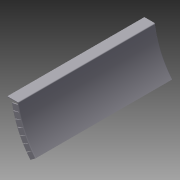
# Autodesk Inventor part: 8 ball ramp
Saved by Autodesk Inventor 2012 (Build 160160000, 160)
## iProperties
Created: 2013-10-24
Part Number: 8 ball ramp
Material: Default
Document SubType Name: Modeling
Designer: Bryce
Density: 1 g/cm^3
Author: Bryce
Autodesk Inventor part; units mm, degrees
ref_plane "YZ Plane" through (0, 0, 0) normal (1, 0, 0) x (0, 1, 0)
ref_plane "XZ Plane" through (0, 0, 0) normal (0, 1, 0) x (-1, 0, 0)
ref_plane "XY Plane" through (0, 0, 0) normal (0, 0, 1) x (1, 0, 0)
sketch "Sketch1" plane through (0, 0, 0) normal (0, 0, 1) x (1, 0, 0)
  line L0 (0, 0) -> (-22.225, 0)
  line L1 (-22.225, 0) -> (-22.225, 1.5875)
  line L2 (-22.225, 1.5875) -> (1.377, 1.5875)
  arc A0 (0, 0) -> (38.1, -85.8654) centre (173.0503, 25.4) ccw
  arc A1 (1.377, 1.5875) -> (39.3249, -84.8555) centre (173.0503, 25.4) ccw
  line L3 (39.3249, -84.8555) -> (38.1, -85.8654)
  dimension "d0" = 1.5875
  dimension "d1" = 22.225
  dimension "d2" = 174.9044
  dimension "d3" = 25.4
  dimension "d4" = 38.1
  dimension "d5" = 1.5875
  constraints: 8 end point, 4 point on circle, 2 centre point, 1 coincident, 1 horizontal, 1 parallel, 1 perpendicular, 1 point on line
  measures "d0" distance of L0.end L1.end
  measures "d1" distance of L0.start L0.end
  measures "d2" radius of A0
  measures "d3" distance from line of A0.centre L0
  measures "d4" horizontal distance of L0.start L3.end
  measures "d5" distance of L3.start L3.end
extrude "Extrusion1" add sketch "Sketch1" along normal blind 298.45
fillet "Fillet1" radius 1.5875 3 edges at (1.377, 1.5875, 149.225) (14.3518, -44.2675, 298.45) (14.3518, -44.2675, 0)
sketch "Sketch2" plane through (0, 0, 298.45) normal (0, 0, 1) x (1, 0, 0)
  arc A0 (0, 0) -> (38.1, -85.8654) centre (173.0503, 25.4) ccw projected
  line L0 (0.4959, -3.175) -> (-11.9499, -5.7034)
  line L1 (-11.9499, -5.7034) -> (-9.4215, -18.1492)
  line L2 (-9.4215, -18.1492) -> (3.0242, -15.6208)
  arc A1 (0.4959, -3.175) -> (3.0242, -15.6208) centre (173.0503, 25.4) ccw
  line L3 (3.1362, -16.0819) -> (-9.084, -19.5399)
  line L4 (-9.084, -19.5399) -> (-5.626, -31.76)
  line L5 (-5.626, -31.76) -> (6.5941, -28.3021)
  arc A2 (3.1362, -16.0819) -> (6.5941, -28.3021) centre (173.0503, 25.4) ccw
  line L6 (6.7404, -28.7535) -> (-5.1848, -33.1214)
  line L7 (-5.1848, -33.1214) -> (-0.8168, -45.0466)
  line L8 (-0.8168, -45.0466) -> (11.1084, -40.6787)
  arc A3 (6.7404, -28.7535) -> (11.1084, -40.6787) centre (173.0503, 25.4) ccw
  line L9 (11.2883, -41.1178) -> (-0.2743, -46.371)
  line L10 (-0.2743, -46.371) -> (4.9788, -57.9336)
  line L11 (4.9788, -57.9336) -> (16.5415, -52.6804)
  arc A4 (11.2883, -41.1178) -> (16.5415, -52.6804) centre (173.0503, 25.4) ccw
  line L12 (16.7539, -53.1047) -> (5.6195, -59.2133)
  line L13 (5.6195, -59.2133) -> (11.728, -70.3477)
  line L14 (11.728, -70.3477) -> (22.8625, -64.2391)
  arc A5 (16.7539, -53.1047) -> (22.8625, -64.2391) centre (173.0503, 25.4) ccw
  line L15 (23.1062, -64.6463) -> (12.4631, -71.5756)
  line L16 (12.4631, -71.5756) -> (19.3925, -82.2186)
  line L17 (19.3925, -82.2186) -> (30.0355, -75.2893)
  arc A6 (23.1062, -64.6463) -> (30.0355, -75.2893) centre (173.0503, 25.4) ccw
  line L18 (30.3092, -75.6769) -> (20.2179, -83.3877)
  line L19 (20.2179, -83.3877) -> (27.9287, -93.479)
  line L20 (27.9287, -93.479) -> (38.02, -85.7682)
  arc A7 (30.3092, -75.6769) -> (38.02, -85.7682) centre (173.0503, 25.4) ccw
  dimension "d16" = 12.7
  dimension "d17" = 3.175
  dimension "d20" = 25.9
  constraints: 42 end point, 15 point on circle, 7 centre point, 2 equal length, 1 coincident, 1 parallel, 1 perpendicular, 55 other
  measures "d16" distance of L0.end L1.end
  measures "d17" vertical distance of L0.start A0.start
extrude "Extrusion2" add sketch "Sketch2" against normal blind 298.45
extrude "Extrusion3" cut sketch "Sketch2" against normal blind 296.8625
extrude "Extrusion4" add sketch "Sketch2" against normal blind 1.5875
body "Solid1"
